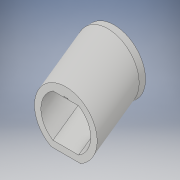
# Autodesk Inventor part: ramp connect both ends
Saved by Autodesk Inventor 2017 (Build 210142000, 142)
## iProperties
Created: 2018-03-06
Part Number: ramp connect both ends
Material: Generic
Document SubType Name: Modeling
Designer: braxtonwright
Density: 1 g/cm^3
Appearance: Default
Author: braxtonwright
Autodesk Inventor part; units mm, degrees
ref_plane "YZ Plane" through (0, 0, 0) normal (1, 0, 0) x (0, 1, 0)
ref_plane "XZ Plane" through (0, 0, 0) normal (0, 1, 0) x (-1, 0, 0)
ref_plane "XY Plane" through (0, 0, 0) normal (0, 0, 1) x (1, 0, 0)
sketch "Sketch1" plane through (0, 0, 0) normal (0, 0, 1) x (1, 0, 0)
  line L0 (-50.8, -84.6667) -> (50.8, -84.6667)
  arc A0 (57.793, -110.0667) -> (-57.793, -110.0667) centre (0, 0) ccw
  arc A1 (-50.8, 84.6667) -> (-50.8, -84.6667) centre (0, 0) ccw
  arc A2 (50.8, -84.6667) -> (50.8, 84.6667) centre (0, 0) ccw
  line L1 (-57.793, -110.0667) -> (57.793, -110.0667)
  line L2 (0, 84.6667) -> (0, 87.8417) construction
  line L3 (-7.4083, 87.8417) -> (7.4083, 87.8417)
  line L4 (-7.4083, 87.8417) -> (-7.4083, 86.2542)
  line L5 (7.4083, 87.8417) -> (7.4083, 86.2542)
  line L6 (0, 84.6667) -> (8.9958, 84.6667) construction
  arc A3 (7.4083, 86.2542) -> (8.9958, 84.6667) centre (8.9958, 86.2542) ccw
  arc A4 (-8.9958, 84.6667) -> (-7.4083, 86.2542) centre (-8.9958, 86.2542) ccw
  line L7 (-50.8, 84.6667) -> (-8.9958, 84.6667)
  line L8 (8.9958, 84.6667) -> (50.8, 84.6667)
  line L9 (0, 84.6667) -> (-8.9958, 84.6667) construction
  line L10 (-6.35, 87.8417) -> (0, 87.8417)
  line L11 (7.4083, 87.8417) -> (-7.4083, 87.8417)
  line L12 (-6.35, 87.8417) -> (-6.35, 86.6178)
  line L13 (-4.1034, 84.646) -> (0, 84.646)
  line L14 (0, 84.646) -> (0, 87.8417) construction
  line L15 (-6.3485, 84.6667) -> (-3.1743, 87.8409) construction
  arc A5 (-3.1736, 84.646) -> (-6.35, 87.8417) centre (-6.3485, 84.6667) ccw construction
  arc A6 (-6.35, 86.6178) -> (-4.1034, 84.646) centre (-4.1034, 86.9117) ccw
  line L16 (6.35, 87.8417) -> (0, 87.8417)
  line L17 (6.35, 87.8417) -> (6.35, 86.6178)
  line L18 (4.1034, 84.646) -> (0, 84.646)
  line L19 (6.3485, 84.6667) -> (3.1743, 87.8409) construction
  arc A7 (6.35, 87.8417) -> (3.1736, 84.646) centre (6.3485, 84.6667) ccw construction
  arc A8 (4.1034, 84.646) -> (6.35, 86.6178) centre (4.1034, 86.9117) ccw
  line L20 (6.35, 87.8417) -> (-6.35, 87.8417)
  dimension "d1" = 101.6
  dimension "d2" = 25.4
  dimension "d34" = 14.8167
  dimension "d35" = 1.5875
  dimension "d36" = 1.5875
  dimension "d38" = 6.35
  dimension "d39" = 3.175
  dimension "d40" = 45
  dimension "d41" = 2.2657
  dimension "d42" = 2.2466
  constraints: 42 end point, 20 point on circle, 11 symmetric about line, 9 centre point, 8 horizontal, 4 coincident, 4 point on line, 2 midpoint, 2 parallel, 2 perpendicular, 2 tangent, 2 vertical, 1 collinear, 3 other
  measures "d1" distance of L7.start L8.end
  measures "d2" distance between parallel lines of L0 L1
  measures "d34" distance of L3.start L5.start
  measures "d35" distance from line of L6.end L5
  measures "d36" radius of A3
  measures "d38" distance of L14.end L10.start
  measures "d39" distance of L10.start L15.start
  measures "d40" angle of L10 L15
  measures "d41" radius of A6
  measures "d42" horizontal distance of L13.start L12.end
extrude "connecction top" add sketch "Sketch1" against normal blind 25.4
extrude "light flat" add sketch "Sketch1" against normal up to surface (25.4 mm away) separate body contours L3 L17 A8 L18 L13 A6 L12
ref_plane "Work Plane2" through (0, 0, 203.2) normal (0, 0, 1) x (1, 0, 0)
sketch "Sketch6" plane through (0, 0, 0) normal (1, 0, 0) x (0, 1, 0)
  line L0 (-110.0667, 0) -> (124.3169, 0) projected
  line L1 (-83.4784, 0) -> (-200.0291, 166.4517)
  point P0 (0, 0)
  dimension "d28" = 203.2
  dimension "d29" = 55
  constraints: 2 end point, 1 point on line
  measures "d28" distance of L1.start L1.end
  measures "d29" angle of L0 L1
sweep "ramp" add profiles "Sketch1" path "Sketch6" bodies 1 path curves L1
sweep "light angle" add profiles "Sketch1" path "Sketch6" separate body path curves L1 contours L3 L17 A8 L18 L13 A6 L12
equation "\"d35\" = 0.5 * d37"
equation "\"d37\" = 3.175"
body "Solid1"
body "Solid2"
body "Solid3"
